Autodesk Inventor part; units mm, degrees
(part 4 of 4)
sketch "Sketch10" plane through (0, 0, 37.211) normal (0, 0, 1) x (1, 0, 0)
  circle A0 centre (33.02, 0) radius 1.778 projected
  circle A1 centre (-33.02, 0) radius 1.778 projected
  circle A2 centre (0, 33.02) radius 1.778 projected
  circle A3 centre (0, -33.02) radius 1.778 projected
  arc A4 (23.7849, -5.4293) -> (23.8053, -5.3393) centre (0, 0) ccw projected
  arc A5 (23.7849, -5.4293) -> (23.9317, -5.7614) centre (24.081, -5.4969) ccw projected
  arc A6 (25.3196, -6.7104) -> (23.9317, -5.7614) centre (19.1245, -14.2809) ccw projected
  arc A7 (25.1433, -7.3435) -> (25.3196, -6.7104) centre (0, 0) ccw projected
  arc A8 (23.4646, -7.4385) -> (25.1433, -7.3435) centre (23.7533, 2.3395) ccw projected
  arc A9 (23.4646, -7.4385) -> (23.1673, -7.6469) centre (23.4557, -7.7421) ccw projected
  arc A10 (23.1382, -7.7345) -> (23.1673, -7.6469) centre (0, 0) ccw projected
  arc A11 (23.1382, -7.7345) -> (23.2518, -8.0793) centre (23.4262, -7.8307) ccw projected
  arc A12 (24.54, -9.1598) -> (23.2518, -8.0793) centre (17.6326, -16.0867) ccw projected
  arc A13 (24.3024, -9.7726) -> (24.54, -9.1598) centre (0, 0) ccw projected
  arc A14 (22.6226, -9.7026) -> (24.3024, -9.7726) centre (23.8682, 0) ccw projected
  arc A15 (22.6226, -9.7026) -> (22.3062, -9.8809) centre (22.5839, -10.0039) ccw projected
  arc A16 (22.2687, -9.9652) -> (22.3062, -9.8809) centre (0, 0) ccw projected
  arc A17 (22.2687, -9.9652) -> (22.3479, -10.3195) centre (22.5459, -10.0892) ccw projected
  arc A18 (23.524, -11.5211) -> (22.3479, -10.3195) centre (15.9709, -17.7375) ccw projected
  arc A19 (23.2275, -12.1076) -> (23.524, -11.5211) centre (0, 0) ccw projected
  arc A20 (21.5626, -11.8733) -> (23.2275, -12.1076) centre (23.7533, -2.3395) ccw projected
  arc A21 (21.5626, -11.8733) -> (21.2303, -12.0197) centre (21.4946, -12.1693) ccw projected
  arc A22 (21.1847, -12.0999) -> (21.2303, -12.0197) centre (0, 0) ccw projected
  arc A23 (21.1847, -12.0999) -> (21.2288, -12.4603) centre (21.4484, -12.2505) ccw projected
  arc A24 (22.2814, -13.7713) -> (21.2288, -12.4603) centre (14.1555, -19.2175) ccw projected
  arc A25 (21.9289, -14.326) -> (22.2814, -13.7713) centre (0, 0) ccw projected
  arc A26 (20.295, -13.9297) -> (21.9289, -14.326) centre (23.4096, -4.6565) ccw projected
  arc A27 (20.295, -13.9297) -> (19.95, -14.0427) centre (20.1983, -14.2175) ccw projected
  arc A28 (19.8967, -14.1181) -> (19.95, -14.0427) centre (0, 0) ccw projected
  arc A29 (19.8967, -14.1181) -> (19.9053, -14.4811) centre (20.1444, -14.2938) ccw projected
  arc A30 (20.8243, -15.889) -> (19.9053, -14.4811) centre (12.2036, -20.5125) ccw projected
  arc A31 (20.4191, -16.4065) -> (20.8243, -15.889) centre (0, 0) ccw projected
  arc A32 (18.8319, -15.8518) -> (20.4191, -16.4065) centre (22.8404, -6.9286) ccw projected
  arc A33 (18.8319, -15.8518) -> (18.4775, -15.9306) centre (18.7075, -16.1289) ccw projected
  arc A34 (18.4171, -16.0003) -> (18.4775, -15.9306) centre (0, 0) ccw projected
  arc A35 (18.4171, -16.0003) -> (18.39, -16.3624) centre (18.6463, -16.1995) ccw projected
  arc A36 (19.1667, -17.8536) -> (18.39, -16.3624) centre (10.1343, -21.6099) ccw projected
  arc A37 (18.7127, -18.3289) -> (19.1667, -17.8536) centre (0, 0) ccw projected
  arc A38 (17.1875, -17.6214) -> (18.7127, -18.3289) centre (22.0513, -9.134) ccw projected
  arc A39 (17.1875, -17.6214) -> (16.827, -17.6649) centre (17.0365, -17.8848) ccw projected
  arc A40 (16.7601, -17.7285) -> (16.827, -17.6649) centre (0, 0) ccw projected
  arc A41 (16.7601, -17.7285) -> (16.6977, -18.0862) centre (16.9687, -17.9492) ccw projected
  arc A42 (17.3244, -19.6463) -> (16.6977, -18.0862) centre (7.9674, -22.4991) ccw projected
  arc A43 (16.826, -20.0748) -> (17.3244, -19.6463) centre (0, 0) ccw projected
  arc A44 (15.3775, -19.2212) -> (16.826, -20.0748) centre (21.0499, -11.2514) ccw projected
  arc A45 (15.3775, -19.2212) -> (15.0145, -19.2292) centre (15.2014, -19.4686) ccw projected
  arc A46 (14.9417, -19.2859) -> (15.0145, -19.2292) centre (0, 0) ccw projected
  arc A47 (14.9417, -19.2859) -> (14.8445, -19.6357) centre (15.1277, -19.5259) ccw projected
  arc A48 (15.3153, -21.2498) -> (14.8445, -19.6357) centre (5.7237, -23.1717) ccw projected
  arc A49 (14.7773, -21.6274) -> (15.3153, -21.2498) centre (0, 0) ccw projected
  arc A50 (13.4195, -20.6359) -> (14.7773, -21.6274) centre (19.8457, -13.2605) ccw projected
  arc A51 (13.4195, -20.6359) -> (13.0574, -20.6083) centre (13.22, -20.8648) ccw projected
  arc A52 (12.9794, -20.6576) -> (13.0574, -20.6083) centre (0, 0) ccw projected
  arc A53 (12.9794, -20.6576) -> (12.8484, -20.9962) centre (13.141, -20.9147) ccw projected
  arc A54 (13.1587, -22.6486) -> (12.8484, -20.9962) centre (3.4249, -23.6212) ccw projected
  arc A55 (12.5863, -22.9716) -> (13.1587, -22.6486) centre (0, 0) ccw projected
  arc A56 (11.3322, -21.8518) -> (12.5863, -22.9716) centre (18.4504, -15.1418) ccw projected
  arc A57 (11.3322, -21.8518) -> (10.9746, -21.7889) centre (11.1112, -22.0602) ccw projected
  arc A58 (10.8921, -21.8303) -> (10.9746, -21.7889) centre (0, 0) ccw projected
  arc A59 (10.8921, -21.8303) -> (10.7286, -22.1544) centre (11.0277, -22.102) ccw projected
  arc A60 (10.8754, -23.8294) -> (10.7286, -22.1544) centre (1.0931, -23.8431) ccw projected
  arc A61 (10.2741, -24.0947) -> (10.8754, -23.8294) centre (0, 0) ccw projected
  arc A62 (9.1358, -22.8574) -> (10.2741, -24.0947) centre (16.8774, -16.8774) ccw projected
  arc A63 (9.1358, -22.8574) -> (8.7861, -22.7597) centre (8.8954, -23.043) ccw projected
  arc A64 (8.6999, -22.7928) -> (8.7861, -22.7597) centre (0, 0) ccw projected
  arc A65 (8.6999, -22.7928) -> (8.5054, -23.0994) centre (8.8082, -23.0765) ccw projected
  arc A66 (8.4873, -24.7806) -> (8.5054, -23.0994) centre (-1.2492, -23.8355) ccw projected
  arc A67 (7.863, -24.9857) -> (8.4873, -24.7806) centre (0, 0) ccw projected
  arc A68 (6.8514, -23.6428) -> (7.863, -24.9857) centre (15.1418, -18.4504) ccw projected
  arc A69 (6.8514, -23.6428) -> (6.5129, -23.5113) centre (6.594, -23.804) ccw projected
  arc A70 (6.4239, -23.5358) -> (6.5129, -23.5113) centre (0, 0) ccw projected
  arc A71 (6.4239, -23.5358) -> (6.2003, -23.8218) centre (6.5039, -23.8287) ccw projected
  arc A72 (6.0176, -25.4932) -> (6.2003, -23.8218) centre (-3.5794, -23.5983) ccw projected
  arc A73 (5.3761, -25.6361) -> (6.0176, -25.4932) centre (0, 0) ccw projected
  arc A74 (4.501, -24.2005) -> (5.3761, -25.6361) centre (13.2605, -19.8457) ccw projected
  arc A75 (4.501, -24.2005) -> (4.177, -24.0365) centre (4.229, -24.3357) ccw projected
  arc A76 (4.0861, -24.0521) -> (4.177, -24.0365) centre (0, 0) ccw projected
  arc A77 (4.0861, -24.0521) -> (3.8355, -24.3148) centre (4.137, -24.3515) ccw projected
  arc A78 (3.4898, -25.9602) -> (3.8355, -24.3148) centre (-5.8752, -23.1338) ccw projected
  arc A79 (2.8374, -26.0396) -> (3.4898, -25.9602) centre (0, 0) ccw projected
  arc A80 (2.1072, -24.5251) -> (2.8374, -26.0396) centre (11.2514, -21.0499) ccw projected
  arc A81 (2.1072, -24.5251) -> (1.8009, -24.3301) centre (1.8234, -24.633) ccw projected
  arc A82 (1.7089, -24.3368) -> (1.8009, -24.3301) centre (0, 0) ccw projected
  arc A83 (1.7089, -24.3368) -> (1.4337, -24.5737) centre (1.7302, -24.6397) ccw projected
  arc A84 (0.9285, -26.1773) -> (1.4337, -24.5737) centre (-8.1145, -22.4465) ccw projected
  arc A85 (0.2714, -26.1923) -> (0.9285, -26.1773) centre (0, 0) ccw projected
  arc A86 (-0.3068, -24.6136) -> (0.2714, -26.1923) centre (9.134, -22.0513) ccw projected
  arc A87 (-0.3068, -24.6136) -> (-0.5925, -24.3895) centre (-0.5999, -24.6931) ccw projected
  arc A88 (-0.6848, -24.3871) -> (-0.5925, -24.3895) centre (0, 0) ccw projected
  arc A89 (-0.6848, -24.3871) -> (-0.9818, -24.5959) centre (-0.6933, -24.6907) ccw projected
  arc A90 (-1.6418, -26.1422) -> (-0.9818, -24.5959) centre (-10.2755, -21.5431) ccw projected
  arc A91 (-2.2972, -26.0928) -> (-1.6418, -26.1422) centre (0, 0) ccw projected
  arc A92 (-2.7179, -24.465) -> (-2.2972, -26.0928) centre (6.9286, -22.8404) ccw projected
  arc A93 (-2.7179, -24.465) -> (-2.9802, -24.214) centre (-3.0173, -24.5154) ccw projected
  arc A94 (-3.0718, -24.2025) -> (-2.9802, -24.214) centre (0, 0) ccw projected
  arc A95 (-3.0718, -24.2025) -> (-3.3879, -24.3812) centre (-3.11, -24.5038) ccw projected
  arc A96 (-4.1963, -25.8554) -> (-3.3879, -24.3812) centre (-12.3376, -20.4322) ccw projected
  arc A97 (-4.8437, -25.742) -> (-4.1963, -25.8554) centre (0, 0) ccw projected
  arc A98 (-5.1028, -24.0808) -> (-4.8437, -25.742) centre (4.6565, -23.4096) ccw projected
  arc A99 (-5.1028, -24.0808) -> (-5.3393, -23.8053) centre (-5.4057, -24.1016) ccw projected
  arc A100 (-5.4293, -23.7849) -> (-5.3393, -23.8053) centre (0, 0) ccw projected
  arc A101 (-5.4293, -23.7849) -> (-5.7614, -23.9317) centre (-5.4969, -24.081) ccw projected
  arc A102 (-6.7104, -25.3196) -> (-5.7614, -23.9317) centre (-14.2809, -19.1245) ccw projected
  arc A103 (-7.3435, -25.1433) -> (-6.7104, -25.3196) centre (0, 0) ccw projected
  arc A104 (-7.4385, -23.4646) -> (-7.3435, -25.1433) centre (2.3395, -23.7533) ccw projected
  arc A105 (-7.4385, -23.4646) -> (-7.6469, -23.1673) centre (-7.7421, -23.4557) ccw projected
  arc A106 (-7.7345, -23.1382) -> (-7.6469, -23.1673) centre (0, 0) ccw projected
  arc A107 (-7.7345, -23.1382) -> (-8.0793, -23.2518) centre (-7.8307, -23.4262) ccw projected
  arc A108 (-9.1598, -24.54) -> (-8.0793, -23.2518) centre (-16.0867, -17.6326) ccw projected
  arc A109 (-9.7726, -24.3024) -> (-9.1598, -24.54) centre (0, 0) ccw projected
  arc A110 (-9.7026, -22.6226) -> (-9.7726, -24.3024) centre (0, -23.8682) ccw projected
  arc A111 (-9.7026, -22.6226) -> (-9.8809, -22.3062) centre (-10.0039, -22.5839) ccw projected
  arc A112 (-9.9652, -22.2687) -> (-9.8809, -22.3062) centre (0, 0) ccw projected
  arc A113 (-9.9652, -22.2687) -> (-10.3195, -22.3479) centre (-10.0892, -22.5459) ccw projected
  arc A114 (-11.5211, -23.524) -> (-10.3195, -22.3479) centre (-17.7375, -15.9709) ccw projected
  arc A115 (-12.1076, -23.2275) -> (-11.5211, -23.524) centre (0, 0) ccw projected
  arc A116 (-11.8733, -21.5626) -> (-12.1076, -23.2275) centre (-2.3395, -23.7533) ccw projected
  arc A117 (-11.8733, -21.5626) -> (-12.0197, -21.2303) centre (-12.1693, -21.4946) ccw projected
  arc A118 (-12.0999, -21.1847) -> (-12.0197, -21.2303) centre (0, 0) ccw projected
  arc A119 (-12.0999, -21.1847) -> (-12.4603, -21.2288) centre (-12.2505, -21.4484) ccw projected
  arc A120 (-13.7713, -22.2814) -> (-12.4603, -21.2288) centre (-19.2175, -14.1555) ccw projected
  arc A121 (-14.326, -21.9289) -> (-13.7713, -22.2814) centre (0, 0) ccw projected
  arc A122 (-13.9297, -20.295) -> (-14.326, -21.9289) centre (-4.6565, -23.4096) ccw projected
  arc A123 (-13.9297, -20.295) -> (-14.0427, -19.95) centre (-14.2175, -20.1983) ccw projected
  arc A124 (-14.1181, -19.8967) -> (-14.0427, -19.95) centre (0, 0) ccw projected
  arc A125 (-14.1181, -19.8967) -> (-14.4811, -19.9053) centre (-14.2938, -20.1444) ccw projected
  arc A126 (-15.889, -20.8243) -> (-14.4811, -19.9053) centre (-20.5125, -12.2036) ccw projected
  arc A127 (-16.4065, -20.4191) -> (-15.889, -20.8243) centre (0, 0) ccw projected
  arc A128 (-15.8518, -18.8319) -> (-16.4065, -20.4191) centre (-6.9286, -22.8404) ccw projected
  arc A129 (-15.8518, -18.8319) -> (-15.9306, -18.4775) centre (-16.1289, -18.7075) ccw projected
  arc A130 (-16.0003, -18.4171) -> (-15.9306, -18.4775) centre (0, 0) ccw projected
  arc A131 (-16.0003, -18.4171) -> (-16.3624, -18.39) centre (-16.1995, -18.6463) ccw projected
  arc A132 (-17.8536, -19.1667) -> (-16.3624, -18.39) centre (-21.6099, -10.1343) ccw projected
  arc A133 (-18.3289, -18.7127) -> (-17.8536, -19.1667) centre (0, 0) ccw projected
  arc A134 (-17.6214, -17.1875) -> (-18.3289, -18.7127) centre (-9.134, -22.0513) ccw projected
  arc A135 (-17.6214, -17.1875) -> (-17.6649, -16.827) centre (-17.8848, -17.0365) ccw projected
  arc A136 (-17.7285, -16.7601) -> (-17.6649, -16.827) centre (0, 0) ccw projected
  arc A137 (-17.7285, -16.7601) -> (-18.0862, -16.6977) centre (-17.9492, -16.9687) ccw projected
  arc A138 (-19.6463, -17.3244) -> (-18.0862, -16.6977) centre (-22.4991, -7.9674) ccw projected
  arc A139 (-20.0748, -16.826) -> (-19.6463, -17.3244) centre (0, 0) ccw projected
  arc A140 (-19.2212, -15.3775) -> (-20.0748, -16.826) centre (-11.2514, -21.0499) ccw projected
  arc A141 (-19.2212, -15.3775) -> (-19.2292, -15.0145) centre (-19.4686, -15.2014) ccw projected
  arc A142 (-19.2859, -14.9417) -> (-19.2292, -15.0145) centre (0, 0) ccw projected
  arc A143 (-19.2859, -14.9417) -> (-19.6357, -14.8445) centre (-19.5259, -15.1277) ccw projected
  arc A144 (-21.2498, -15.3153) -> (-19.6357, -14.8445) centre (-23.1717, -5.7237) ccw projected
  arc A145 (-21.6274, -14.7773) -> (-21.2498, -15.3153) centre (0, 0) ccw projected
  arc A146 (-20.6359, -13.4195) -> (-21.6274, -14.7773) centre (-13.2605, -19.8457) ccw projected
  arc A147 (-20.6359, -13.4195) -> (-20.6083, -13.0574) centre (-20.8648, -13.22) ccw projected
  arc A148 (-20.6576, -12.9794) -> (-20.6083, -13.0574) centre (0, 0) ccw projected
  arc A149 (-20.6576, -12.9794) -> (-20.9962, -12.8484) centre (-20.9147, -13.141) ccw projected
  arc A150 (-22.6486, -13.1587) -> (-20.9962, -12.8484) centre (-23.6212, -3.4249) ccw projected
  arc A151 (-22.9716, -12.5863) -> (-22.6486, -13.1587) centre (0, 0) ccw projected
  arc A152 (-21.8518, -11.3322) -> (-22.9716, -12.5863) centre (-15.1418, -18.4504) ccw projected
  arc A153 (-21.8518, -11.3322) -> (-21.7889, -10.9746) centre (-22.0602, -11.1112) ccw projected
  arc A154 (-21.8303, -10.8921) -> (-21.7889, -10.9746) centre (0, 0) ccw projected
  arc A155 (-21.8303, -10.8921) -> (-22.1544, -10.7286) centre (-22.102, -11.0277) ccw projected
  arc A156 (-23.8294, -10.8754) -> (-22.1544, -10.7286) centre (-23.8431, -1.0931) ccw projected
  arc A157 (-24.0947, -10.2741) -> (-23.8294, -10.8754) centre (0, 0) ccw projected
  arc A158 (-22.8574, -9.1358) -> (-24.0947, -10.2741) centre (-16.8774, -16.8774) ccw projected
  arc A159 (-22.8574, -9.1358) -> (-22.7597, -8.7861) centre (-23.043, -8.8954) ccw projected
  arc A160 (-22.7928, -8.6999) -> (-22.7597, -8.7861) centre (0, 0) ccw projected
  arc A161 (-22.7928, -8.6999) -> (-23.0994, -8.5054) centre (-23.0765, -8.8082) ccw projected
  arc A162 (-24.7806, -8.4873) -> (-23.0994, -8.5054) centre (-23.8355, 1.2492) ccw projected
  arc A163 (-24.9857, -7.863) -> (-24.7806, -8.4873) centre (0, 0) ccw projected
  arc A164 (-23.6428, -6.8514) -> (-24.9857, -7.863) centre (-18.4504, -15.1418) ccw projected
  arc A165 (-23.6428, -6.8514) -> (-23.5113, -6.5129) centre (-23.804, -6.594) ccw projected
  arc A166 (-23.5358, -6.4239) -> (-23.5113, -6.5129) centre (0, 0) ccw projected
  arc A167 (-23.5358, -6.4239) -> (-23.8218, -6.2003) centre (-23.8287, -6.5039) ccw projected
  arc A168 (-25.4932, -6.0176) -> (-23.8218, -6.2003) centre (-23.5983, 3.5794) ccw projected
  arc A169 (-25.6361, -5.3761) -> (-25.4932, -6.0176) centre (0, 0) ccw projected
  arc A170 (-24.2005, -4.501) -> (-25.6361, -5.3761) centre (-19.8457, -13.2605) ccw projected
  arc A171 (-24.2005, -4.501) -> (-24.0365, -4.177) centre (-24.3357, -4.229) ccw projected
  arc A172 (-24.0521, -4.0861) -> (-24.0365, -4.177) centre (0, 0) ccw projected
  arc A173 (-24.0521, -4.0861) -> (-24.3148, -3.8355) centre (-24.3515, -4.137) ccw projected
  arc A174 (-25.9602, -3.4898) -> (-24.3148, -3.8355) centre (-23.1338, 5.8752) ccw projected
  arc A175 (-26.0396, -2.8374) -> (-25.9602, -3.4898) centre (0, 0) ccw projected
  arc A176 (-24.5251, -2.1072) -> (-26.0396, -2.8374) centre (-21.0499, -11.2514) ccw projected
  arc A177 (-24.5251, -2.1072) -> (-24.3301, -1.8009) centre (-24.633, -1.8234) ccw projected
  arc A178 (-24.3368, -1.7089) -> (-24.3301, -1.8009) centre (0, 0) ccw projected
  arc A179 (-24.3368, -1.7089) -> (-24.5737, -1.4337) centre (-24.6397, -1.7302) ccw projected
  arc A180 (-26.1773, -0.9285) -> (-24.5737, -1.4337) centre (-22.4465, 8.1145) ccw projected
  arc A181 (-26.1923, -0.2714) -> (-26.1773, -0.9285) centre (0, 0) ccw projected
  arc A182 (-24.6136, 0.3068) -> (-26.1923, -0.2714) centre (-22.0513, -9.134) ccw projected
  arc A183 (-24.6136, 0.3068) -> (-24.3895, 0.5925) centre (-24.6931, 0.5999) ccw projected
  arc A184 (-24.3871, 0.6848) -> (-24.3895, 0.5925) centre (0, 0) ccw projected
  arc A185 (-24.3871, 0.6848) -> (-24.5959, 0.9818) centre (-24.6907, 0.6933) ccw projected
  arc A186 (-26.1422, 1.6418) -> (-24.5959, 0.9818) centre (-21.5431, 10.2755) ccw projected
  arc A187 (-26.0928, 2.2972) -> (-26.1422, 1.6418) centre (0, 0) ccw projected
  arc A188 (-24.465, 2.7179) -> (-26.0928, 2.2972) centre (-22.8404, -6.9286) ccw projected
  arc A189 (-24.465, 2.7179) -> (-24.214, 2.9802) centre (-24.5154, 3.0173) ccw projected
  arc A190 (-24.2025, 3.0718) -> (-24.214, 2.9802) centre (0, 0) ccw projected
  arc A191 (-24.2025, 3.0718) -> (-24.3812, 3.3879) centre (-24.5038, 3.11) ccw projected
  arc A192 (-25.8554, 4.1963) -> (-24.3812, 3.3879) centre (-20.4322, 12.3376) ccw projected
  arc A193 (-25.742, 4.8437) -> (-25.8554, 4.1963) centre (0, 0) ccw projected
  arc A194 (-24.0808, 5.1028) -> (-25.742, 4.8437) centre (-23.4096, -4.6565) ccw projected
  arc A195 (-24.0808, 5.1028) -> (-23.8053, 5.3393) centre (-24.1016, 5.4057) ccw projected
  arc A196 (-23.7849, 5.4293) -> (-23.8053, 5.3393) centre (0, 0) ccw projected
  arc A197 (-23.7849, 5.4293) -> (-23.9317, 5.7614) centre (-24.081, 5.4969) ccw projected
  arc A198 (-25.3196, 6.7104) -> (-23.9317, 5.7614) centre (-19.1245, 14.2809) ccw projected
  arc A199 (-25.1433, 7.3435) -> (-25.3196, 6.7104) centre (0, 0) ccw projected
  arc A200 (-23.4646, 7.4385) -> (-25.1433, 7.3435) centre (-23.7533, -2.3395) ccw projected
  arc A201 (-23.4646, 7.4385) -> (-23.1673, 7.6469) centre (-23.4557, 7.7421) ccw projected
  arc A202 (-23.1382, 7.7345) -> (-23.1673, 7.6469) centre (0, 0) ccw projected
  arc A203 (-23.1382, 7.7345) -> (-23.2518, 8.0793) centre (-23.4262, 7.8307) ccw projected
  arc A204 (-24.54, 9.1598) -> (-23.2518, 8.0793) centre (-17.6326, 16.0867) ccw projected
  arc A205 (-24.3024, 9.7726) -> (-24.54, 9.1598) centre (0, 0) ccw projected
  arc A206 (-22.6226, 9.7026) -> (-24.3024, 9.7726) centre (-23.8682, 0) ccw projected
  arc A207 (-22.6226, 9.7026) -> (-22.3062, 9.8809) centre (-22.5839, 10.0039) ccw projected
  arc A208 (-22.2687, 9.9652) -> (-22.3062, 9.8809) centre (0, 0) ccw projected
  arc A209 (-22.2687, 9.9652) -> (-22.3479, 10.3195) centre (-22.5459, 10.0892) ccw projected
  arc A210 (-23.524, 11.5211) -> (-22.3479, 10.3195) centre (-15.9709, 17.7375) ccw projected
  arc A211 (-23.2275, 12.1076) -> (-23.524, 11.5211) centre (0, 0) ccw projected
  arc A212 (-21.5626, 11.8733) -> (-23.2275, 12.1076) centre (-23.7533, 2.3395) ccw projected
  arc A213 (-21.5626, 11.8733) -> (-21.2303, 12.0197) centre (-21.4946, 12.1693) ccw projected
  arc A214 (-21.1847, 12.0999) -> (-21.2303, 12.0197) centre (0, 0) ccw projected
  arc A215 (-21.1847, 12.0999) -> (-21.2288, 12.4603) centre (-21.4484, 12.2505) ccw projected
  arc A216 (-22.2814, 13.7713) -> (-21.2288, 12.4603) centre (-14.1555, 19.2175) ccw projected
  arc A217 (-21.9289, 14.326) -> (-22.2814, 13.7713) centre (0, 0) ccw projected
  arc A218 (-20.295, 13.9297) -> (-21.9289, 14.326) centre (-23.4096, 4.6565) ccw projected
  arc A219 (-20.295, 13.9297) -> (-19.95, 14.0427) centre (-20.1983, 14.2175) ccw projected
  arc A220 (-19.8967, 14.1181) -> (-19.95, 14.0427) centre (0, 0) ccw projected
  arc A221 (-19.8967, 14.1181) -> (-19.9053, 14.4811) centre (-20.1444, 14.2938) ccw projected
  arc A222 (-20.8243, 15.889) -> (-19.9053, 14.4811) centre (-12.2036, 20.5125) ccw projected
  arc A223 (-20.4191, 16.4065) -> (-20.8243, 15.889) centre (0, 0) ccw projected
  arc A224 (-18.8319, 15.8518) -> (-20.4191, 16.4065) centre (-22.8404, 6.9286) ccw projected
  arc A225 (-18.8319, 15.8518) -> (-18.4775, 15.9306) centre (-18.7075, 16.1289) ccw projected
  arc A226 (-18.4171, 16.0003) -> (-18.4775, 15.9306) centre (0, 0) ccw projected
  arc A227 (-18.4171, 16.0003) -> (-18.39, 16.3624) centre (-18.6463, 16.1995) ccw projected
  arc A228 (-19.1667, 17.8536) -> (-18.39, 16.3624) centre (-10.1343, 21.6099) ccw projected
  arc A229 (-18.7127, 18.3289) -> (-19.1667, 17.8536) centre (0, 0) ccw projected
  arc A230 (-17.1875, 17.6214) -> (-18.7127, 18.3289) centre (-22.0513, 9.134) ccw projected
  arc A231 (-17.1875, 17.6214) -> (-16.827, 17.6649) centre (-17.0365, 17.8848) ccw projected
  arc A232 (-16.7601, 17.7285) -> (-16.827, 17.6649) centre (0, 0) ccw projected
  arc A233 (-16.7601, 17.7285) -> (-16.6977, 18.0862) centre (-16.9687, 17.9492) ccw projected
  arc A234 (-17.3244, 19.6463) -> (-16.6977, 18.0862) centre (-7.9674, 22.4991) ccw projected
  arc A235 (-16.826, 20.0748) -> (-17.3244, 19.6463) centre (0, 0) ccw projected
  arc A236 (-15.3775, 19.2212) -> (-16.826, 20.0748) centre (-21.0499, 11.2514) ccw projected
  arc A237 (-15.3775, 19.2212) -> (-15.0145, 19.2292) centre (-15.2014, 19.4686) ccw projected
  arc A238 (-14.9417, 19.2859) -> (-15.0145, 19.2292) centre (0, 0) ccw projected
  arc A239 (-14.9417, 19.2859) -> (-14.8445, 19.6357) centre (-15.1277, 19.5259) ccw projected
  arc A240 (-15.3153, 21.2498) -> (-14.8445, 19.6357) centre (-5.7237, 23.1717) ccw projected
  arc A241 (-14.7773, 21.6274) -> (-15.3153, 21.2498) centre (0, 0) ccw projected
  arc A242 (-13.4195, 20.6359) -> (-14.7773, 21.6274) centre (-19.8457, 13.2605) ccw projected
  arc A243 (-13.4195, 20.6359) -> (-13.0574, 20.6083) centre (-13.22, 20.8648) ccw projected
  arc A244 (-12.9794, 20.6576) -> (-13.0574, 20.6083) centre (0, 0) ccw projected
  arc A245 (-12.9794, 20.6576) -> (-12.8484, 20.9962) centre (-13.141, 20.9147) ccw projected
  arc A246 (-13.1587, 22.6486) -> (-12.8484, 20.9962) centre (-3.4249, 23.6212) ccw projected
  arc A247 (-12.5863, 22.9716) -> (-13.1587, 22.6486) centre (0, 0) ccw projected
  arc A248 (-11.3322, 21.8518) -> (-12.5863, 22.9716) centre (-18.4504, 15.1418) ccw projected
  arc A249 (-11.3322, 21.8518) -> (-10.9746, 21.7889) centre (-11.1112, 22.0602) ccw projected
  arc A250 (-10.8921, 21.8303) -> (-10.9746, 21.7889) centre (0, 0) ccw projected
  arc A251 (-10.8921, 21.8303) -> (-10.7286, 22.1544) centre (-11.0277, 22.102) ccw projected
  arc A252 (-10.8754, 23.8294) -> (-10.7286, 22.1544) centre (-1.0931, 23.8431) ccw projected
  arc A253 (-10.2741, 24.0947) -> (-10.8754, 23.8294) centre (0, 0) ccw projected
  arc A254 (-9.1358, 22.8574) -> (-10.2741, 24.0947) centre (-16.8774, 16.8774) ccw projected
  arc A255 (-9.1358, 22.8574) -> (-8.7861, 22.7597) centre (-8.8954, 23.043) ccw projected
  arc A256 (-8.6999, 22.7928) -> (-8.7861, 22.7597) centre (0, 0) ccw projected
  arc A257 (-8.6999, 22.7928) -> (-8.5054, 23.0994) centre (-8.8082, 23.0765) ccw projected
  arc A258 (-8.4873, 24.7806) -> (-8.5054, 23.0994) centre (1.2492, 23.8355) ccw projected
  arc A259 (-7.863, 24.9857) -> (-8.4873, 24.7806) centre (0, 0) ccw projected
  arc A260 (-6.8514, 23.6428) -> (-7.863, 24.9857) centre (-15.1418, 18.4504) ccw projected
  arc A261 (-6.8514, 23.6428) -> (-6.5129, 23.5113) centre (-6.594, 23.804) ccw projected
  arc A262 (-6.4239, 23.5358) -> (-6.5129, 23.5113) centre (0, 0) ccw projected
  arc A263 (-6.4239, 23.5358) -> (-6.2003, 23.8218) centre (-6.5039, 23.8287) ccw projected
  arc A264 (-6.0176, 25.4932) -> (-6.2003, 23.8218) centre (3.5794, 23.5983) ccw projected
  arc A265 (-5.3761, 25.6361) -> (-6.0176, 25.4932) centre (0, 0) ccw projected
  arc A266 (-4.501, 24.2005) -> (-5.3761, 25.6361) centre (-13.2605, 19.8457) ccw projected
  arc A267 (-4.501, 24.2005) -> (-4.177, 24.0365) centre (-4.229, 24.3357) ccw projected
  arc A268 (-4.0861, 24.0521) -> (-4.177, 24.0365) centre (0, 0) ccw projected
  arc A269 (-4.0861, 24.0521) -> (-3.8355, 24.3148) centre (-4.137, 24.3515) ccw projected
  arc A270 (-3.4898, 25.9602) -> (-3.8355, 24.3148) centre (5.8752, 23.1338) ccw projected
  arc A271 (-2.8374, 26.0396) -> (-3.4898, 25.9602) centre (0, 0) ccw projected
  arc A272 (-2.1072, 24.5251) -> (-2.8374, 26.0396) centre (-11.2514, 21.0499) ccw projected
  arc A273 (-2.1072, 24.5251) -> (-1.8009, 24.3301) centre (-1.8234, 24.633) ccw projected
  arc A274 (-1.7089, 24.3368) -> (-1.8009, 24.3301) centre (0, 0) ccw projected
  arc A275 (-1.7089, 24.3368) -> (-1.4337, 24.5737) centre (-1.7302, 24.6397) ccw projected
  arc A276 (-0.9285, 26.1773) -> (-1.4337, 24.5737) centre (8.1145, 22.4465) ccw projected
  arc A277 (-0.2714, 26.1923) -> (-0.9285, 26.1773) centre (0, 0) ccw projected
  arc A278 (0.3068, 24.6136) -> (-0.2714, 26.1923) centre (-9.134, 22.0513) ccw projected
  arc A279 (0.3068, 24.6136) -> (0.5925, 24.3895) centre (0.5999, 24.6931) ccw projected
  arc A280 (0.6848, 24.3871) -> (0.5925, 24.3895) centre (0, 0) ccw projected
  arc A281 (0.6848, 24.3871) -> (0.9818, 24.5959) centre (0.6933, 24.6907) ccw projected
  arc A282 (1.6418, 26.1422) -> (0.9818, 24.5959) centre (10.2755, 21.5431) ccw projected
  arc A283 (2.2972, 26.0928) -> (1.6418, 26.1422) centre (0, 0) ccw projected
  arc A284 (2.7179, 24.465) -> (2.2972, 26.0928) centre (-6.9286, 22.8404) ccw projected
  arc A285 (2.7179, 24.465) -> (2.9802, 24.214) centre (3.0173, 24.5154) ccw projected
  arc A286 (3.0718, 24.2025) -> (2.9802, 24.214) centre (0, 0) ccw projected
  arc A287 (3.0718, 24.2025) -> (3.3879, 24.3812) centre (3.11, 24.5038) ccw projected
  arc A288 (4.1963, 25.8554) -> (3.3879, 24.3812) centre (12.3376, 20.4322) ccw projected
  arc A289 (4.8437, 25.742) -> (4.1963, 25.8554) centre (0, 0) ccw projected
  arc A290 (5.1028, 24.0808) -> (4.8437, 25.742) centre (-4.6565, 23.4096) ccw projected
  arc A291 (5.1028, 24.0808) -> (5.3393, 23.8053) centre (5.4057, 24.1016) ccw projected
  arc A292 (5.4293, 23.7849) -> (5.3393, 23.8053) centre (0, 0) ccw projected
  arc A293 (5.4293, 23.7849) -> (5.7614, 23.9317) centre (5.4969, 24.081) ccw projected
  arc A294 (6.7104, 25.3196) -> (5.7614, 23.9317) centre (14.2809, 19.1245) ccw projected
  arc A295 (7.3435, 25.1433) -> (6.7104, 25.3196) centre (0, 0) ccw projected
  arc A296 (7.4385, 23.4646) -> (7.3435, 25.1433) centre (-2.3395, 23.7533) ccw projected
  arc A297 (7.4385, 23.4646) -> (7.6469, 23.1673) centre (7.7421, 23.4557) ccw projected
  arc A298 (7.7345, 23.1382) -> (7.6469, 23.1673) centre (0, 0) ccw projected
  arc A299 (7.7345, 23.1382) -> (8.0793, 23.2518) centre (7.8307, 23.4262) ccw projected
  arc A300 (9.1598, 24.54) -> (8.0793, 23.2518) centre (16.0867, 17.6326) ccw projected
  arc A301 (9.7726, 24.3024) -> (9.1598, 24.54) centre (0, 0) ccw projected
  arc A302 (9.7026, 22.6226) -> (9.7726, 24.3024) centre (0, 23.8682) ccw projected
  arc A303 (9.7026, 22.6226) -> (9.8809, 22.3062) centre (10.0039, 22.5839) ccw projected
  arc A304 (9.9652, 22.2687) -> (9.8809, 22.3062) centre (0, 0) ccw projected
  arc A305 (9.9652, 22.2687) -> (10.3195, 22.3479) centre (10.0892, 22.5459) ccw projected
  arc A306 (11.5211, 23.524) -> (10.3195, 22.3479) centre (17.7375, 15.9709) ccw projected
  arc A307 (12.1076, 23.2275) -> (11.5211, 23.524) centre (0, 0) ccw projected
  arc A308 (11.8733, 21.5626) -> (12.1076, 23.2275) centre (2.3395, 23.7533) ccw projected
  arc A309 (11.8733, 21.5626) -> (12.0197, 21.2303) centre (12.1693, 21.4946) ccw projected
  arc A310 (12.0999, 21.1847) -> (12.0197, 21.2303) centre (0, 0) ccw projected
  arc A311 (12.0999, 21.1847) -> (12.4603, 21.2288) centre (12.2505, 21.4484) ccw projected
  arc A312 (13.7713, 22.2814) -> (12.4603, 21.2288) centre (19.2175, 14.1555) ccw projected
  arc A313 (14.326, 21.9289) -> (13.7713, 22.2814) centre (0, 0) ccw projected
  arc A314 (13.9297, 20.295) -> (14.326, 21.9289) centre (4.6565, 23.4096) ccw projected
  arc A315 (13.9297, 20.295) -> (14.0427, 19.95) centre (14.2175, 20.1983) ccw projected
  arc A316 (14.1181, 19.8967) -> (14.0427, 19.95) centre (0, 0) ccw projected
  arc A317 (14.1181, 19.8967) -> (14.4811, 19.9053) centre (14.2938, 20.1444) ccw projected
  arc A318 (15.889, 20.8243) -> (14.4811, 19.9053) centre (20.5125, 12.2036) ccw projected
  arc A319 (16.4065, 20.4191) -> (15.889, 20.8243) centre (0, 0) ccw projected
  arc A320 (15.8518, 18.8319) -> (16.4065, 20.4191) centre (6.9286, 22.8404) ccw projected
  arc A321 (15.8518, 18.8319) -> (15.9306, 18.4775) centre (16.1289, 18.7075) ccw projected
  arc A322 (16.0003, 18.4171) -> (15.9306, 18.4775) centre (0, 0) ccw projected
  arc A323 (16.0003, 18.4171) -> (16.3624, 18.39) centre (16.1995, 18.6463) ccw projected
  arc A324 (17.8536, 19.1667) -> (16.3624, 18.39) centre (21.6099, 10.1343) ccw projected
  arc A325 (18.3289, 18.7127) -> (17.8536, 19.1667) centre (0, 0) ccw projected
  arc A326 (17.6214, 17.1875) -> (18.3289, 18.7127) centre (9.134, 22.0513) ccw projected
  arc A327 (17.6214, 17.1875) -> (17.6649, 16.827) centre (17.8848, 17.0365) ccw projected
  arc A328 (17.7285, 16.7601) -> (17.6649, 16.827) centre (0, 0) ccw projected
  arc A329 (17.7285, 16.7601) -> (18.0862, 16.6977) centre (17.9492, 16.9687) ccw projected
  arc A330 (19.6463, 17.3244) -> (18.0862, 16.6977) centre (22.4991, 7.9674) ccw projected
  arc A331 (20.0748, 16.826) -> (19.6463, 17.3244) centre (0, 0) ccw projected
  arc A332 (19.2212, 15.3775) -> (20.0748, 16.826) centre (11.2514, 21.0499) ccw projected
  arc A333 (19.2212, 15.3775) -> (19.2292, 15.0145) centre (19.4686, 15.2014) ccw projected
  arc A334 (19.2859, 14.9417) -> (19.2292, 15.0145) centre (0, 0) ccw projected
  arc A335 (19.2859, 14.9417) -> (19.6357, 14.8445) centre (19.5259, 15.1277) ccw projected
  arc A336 (21.2498, 15.3153) -> (19.6357, 14.8445) centre (23.1717, 5.7237) ccw projected
  arc A337 (21.6274, 14.7773) -> (21.2498, 15.3153) centre (0, 0) ccw projected
  arc A338 (20.6359, 13.4195) -> (21.6274, 14.7773) centre (13.2605, 19.8457) ccw projected
  arc A339 (20.6359, 13.4195) -> (20.6083, 13.0574) centre (20.8648, 13.22) ccw projected
  arc A340 (20.6576, 12.9794) -> (20.6083, 13.0574) centre (0, 0) ccw projected
  arc A341 (20.6576, 12.9794) -> (20.9962, 12.8484) centre (20.9147, 13.141) ccw projected
  arc A342 (22.6486, 13.1587) -> (20.9962, 12.8484) centre (23.6212, 3.4249) ccw projected
  arc A343 (22.9716, 12.5863) -> (22.6486, 13.1587) centre (0, 0) ccw projected
  arc A344 (21.8518, 11.3322) -> (22.9716, 12.5863) centre (15.1418, 18.4504) ccw projected
  arc A345 (21.8518, 11.3322) -> (21.7889, 10.9746) centre (22.0602, 11.1112) ccw projected
  arc A346 (21.8303, 10.8921) -> (21.7889, 10.9746) centre (0, 0) ccw projected
  arc A347 (21.8303, 10.8921) -> (22.1544, 10.7286) centre (22.102, 11.0277) ccw projected
  arc A348 (23.8294, 10.8754) -> (22.1544, 10.7286) centre (23.8431, 1.0931) ccw projected
  arc A349 (24.0947, 10.2741) -> (23.8294, 10.8754) centre (0, 0) ccw projected
  arc A350 (22.8574, 9.1358) -> (24.0947, 10.2741) centre (16.8774, 16.8774) ccw projected
  arc A351 (22.8574, 9.1358) -> (22.7597, 8.7861) centre (23.043, 8.8954) ccw projected
  arc A352 (22.7928, 8.6999) -> (22.7597, 8.7861) centre (0, 0) ccw projected
  arc A353 (22.7928, 8.6999) -> (23.0994, 8.5054) centre (23.0765, 8.8082) ccw projected
  arc A354 (24.7806, 8.4873) -> (23.0994, 8.5054) centre (23.8355, -1.2492) ccw projected
  arc A355 (24.9857, 7.863) -> (24.7806, 8.4873) centre (0, 0) ccw projected
  arc A356 (23.6428, 6.8514) -> (24.9857, 7.863) centre (18.4504, 15.1418) ccw projected
  arc A357 (23.6428, 6.8514) -> (23.5113, 6.5129) centre (23.804, 6.594) ccw projected
  arc A358 (23.5358, 6.4239) -> (23.5113, 6.5129) centre (0, 0) ccw projected
  arc A359 (23.5358, 6.4239) -> (23.8218, 6.2003) centre (23.8287, 6.5039) ccw projected
  arc A360 (25.4932, 6.0176) -> (23.8218, 6.2003) centre (23.5983, -3.5794) ccw projected
  arc A361 (25.6361, 5.3761) -> (25.4932, 6.0176) centre (0, 0) ccw projected
  arc A362 (24.2005, 4.501) -> (25.6361, 5.3761) centre (19.8457, 13.2605) ccw projected
  arc A363 (24.2005, 4.501) -> (24.0365, 4.177) centre (24.3357, 4.229) ccw projected
  arc A364 (24.0521, 4.0861) -> (24.0365, 4.177) centre (0, 0) ccw projected
  arc A365 (24.0521, 4.0861) -> (24.3148, 3.8355) centre (24.3515, 4.137) ccw projected
  arc A366 (25.9602, 3.4898) -> (24.3148, 3.8355) centre (23.1338, -5.8752) ccw projected
  arc A367 (26.0396, 2.8374) -> (25.9602, 3.4898) centre (0, 0) ccw projected
  arc A368 (24.5251, 2.1072) -> (26.0396, 2.8374) centre (21.0499, 11.2514) ccw projected
  arc A369 (24.5251, 2.1072) -> (24.3301, 1.8009) centre (24.633, 1.8234) ccw projected
  arc A370 (24.3368, 1.7089) -> (24.3301, 1.8009) centre (0, 0) ccw projected
  arc A371 (24.3368, 1.7089) -> (24.5737, 1.4337) centre (24.6397, 1.7302) ccw projected
  arc A372 (26.1773, 0.9285) -> (24.5737, 1.4337) centre (22.4465, -8.1145) ccw projected
  arc A373 (26.1923, 0.2714) -> (26.1773, 0.9285) centre (0, 0) ccw projected
  arc A374 (24.6136, -0.3068) -> (26.1923, 0.2714) centre (22.0513, 9.134) ccw projected
  arc A375 (24.6136, -0.3068) -> (24.3895, -0.5925) centre (24.6931, -0.5999) ccw projected
  arc A376 (24.3871, -0.6848) -> (24.3895, -0.5925) centre (0, 0) ccw projected
  arc A377 (24.3871, -0.6848) -> (24.5959, -0.9818) centre (24.6907, -0.6933) ccw projected
  arc A378 (26.1422, -1.6418) -> (24.5959, -0.9818) centre (21.5431, -10.2755) ccw projected
  arc A379 (26.0928, -2.2972) -> (26.1422, -1.6418) centre (0, 0) ccw projected
  arc A380 (24.465, -2.7179) -> (26.0928, -2.2972) centre (22.8404, 6.9286) ccw projected
  arc A381 (24.465, -2.7179) -> (24.214, -2.9802) centre (24.5154, -3.0173) ccw projected
  arc A382 (24.2025, -3.0718) -> (24.214, -2.9802) centre (0, 0) ccw projected
  arc A383 (24.2025, -3.0718) -> (24.3812, -3.3879) centre (24.5038, -3.11) ccw projected
  arc A384 (25.8554, -4.1963) -> (24.3812, -3.3879) centre (20.4322, -12.3376) ccw projected
  arc A385 (25.742, -4.8437) -> (25.8554, -4.1963) centre (0, 0) ccw projected
  arc A386 (24.0808, -5.1028) -> (25.742, -4.8437) centre (23.4096, 4.6565) ccw projected
  arc A387 (24.0808, -5.1028) -> (23.8053, -5.3393) centre (24.1016, -5.4057) ccw projected
  arc A388 (29.1925, 4.0714) -> (4.0714, 29.1925) centre (0, 0) ccw projected
  arc A389 (4.0714, 29.1925) -> (-4.0714, 29.1925) centre (0, 33.02) ccw projected
  arc A390 (-4.0714, 29.1925) -> (-29.1925, 4.0714) centre (0, 0) ccw projected
  arc A391 (-29.1925, 4.0714) -> (-29.1925, -4.0714) centre (-33.02, 0) ccw projected
  arc A392 (-29.1925, -4.0714) -> (-4.0714, -29.1925) centre (0, 0) ccw projected
  arc A393 (-4.0714, -29.1925) -> (4.0714, -29.1925) centre (0, -33.02) ccw projected
  arc A394 (4.0714, -29.1925) -> (29.1925, -4.0714) centre (0, 0) ccw projected
  arc A395 (29.1925, -4.0714) -> (29.1925, 4.0714) centre (33.02, 0) ccw projected
  point P0 (0, 0)
fillet "Fillet1" radius 3.175 8 edges at (-4.0714, 29.1925, 30.861) (-29.1925, 4.0714, 30.861) (-29.1925, -4.0714, 30.861) (-4.0714, -29.1925, 30.861) (4.0714, -29.1925, 30.861) (29.1925, -4.0714, 30.861) (29.1925, 4.0714, 30.861) (4.0714, 29.1925, 30.861)
body "Solid1"
